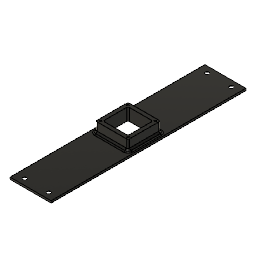
Foosball Table with Camera Stand (Autodesk Fusion 360 archive; units mm, degrees)
design "Camera Holder Middle"
Autodesk Fusion 360 part; units mm, degrees
note: some values were not read from the file. Chosen so that the rebuilt part matches the saved one: which bodies a step acts on; which face or edge a step refers to. Set by a fixed rule: which sketch regions a step uses.
(part 1 of 2)
sketch "Sketch1" plane through (0, 0, 0) normal (0, 0, 1) x (1, 0, 0)
  line L0 (-120.55, 25.4) -> (120.65, 25.4)
  line L1 (120.65, 25.4) -> (120.65, -25.4)
  line L2 (120.65, -25.4) -> (-120.55, -25.4)
  line L3 (-120.55, -25.4) -> (-120.55, 25.4)
  dimension "d3" = 241.2
  dimension "d4" = 50.8
  dimension "d5" = 25.4
  dimension "d6" = 120.65
  constraint horizontal L0
  constraint vertical L1
  constraint horizontal L2
  constraint vertical L3
  measures "d3" distance of L1 L3
  measures "d4" distance of L0 L2
  measures "d5" distance of origin L2
  measures "d6" distance of origin L1
extrude "Extrude1" add sketch "Sketch1" along normal blind 2.5
sketch "Sketch2" plane through (0, 0, 2.5) normal (0, 0, 1) x (-1, 0, 0)
  line L0 (120.55, 25.4) -> (-120.65, 25.4)
  line L1 (-120.65, 25.4) -> (-120.65, -25.4)
  line L2 (-120.65, -25.4) -> (120.55, -25.4)
  line L3 (120.55, -25.4) -> (120.55, 25.4)
  line L4 (13.4, -15.4) -> (-13.4, -15.4)
  line L5 (-15.4, -13.4) -> (-15.4, 13.4)
  line L6 (-13.4, 15.4) -> (13.4, 15.4)
  line L7 (15.4, 13.4) -> (15.4, -13.4)
  arc A0 (13.4, -15.4) -> (15.4, -13.4) centre (13.4, -13.4) ccw
  arc A1 (-15.4, -13.4) -> (-13.4, -15.4) centre (-13.4, -13.4) ccw
  arc A2 (-13.4, 15.4) -> (-15.4, 13.4) centre (-13.4, 13.4) ccw
  arc A3 (15.4, 13.4) -> (13.4, 15.4) centre (13.4, 13.4) ccw
  dimension "d7" = 30.8
  dimension "d8" = 30.8
  dimension "d9" = 15.4
  dimension "d10" = 15.4
  dimension "d11" = 2
  constraint horizontal L4
  constraint vertical L5
  constraint horizontal L6
  constraint vertical L7
  constraint tangent L4 A0
  constraint tangent L7 A0
  constraint tangent L4 A1
  constraint tangent L5 A1
  constraint equal A0 A1
  constraint tangent L5 A2
  constraint tangent L6 A2
  constraint equal A0 A2
  constraint tangent L6 A3
  constraint tangent L7 A3
  constraint equal A0 A3
  measures "d7" distance of L5 L7
  measures "d8" distance of L4 L6
  measures "d9" distance of origin L5
  measures "d10" distance of origin L4
  measures "d11" radius of A0
extrude "Extrude2" cut sketch "Sketch2" against normal blind 2.5 contours L4 L5 L6 L7 A0 A1 A2 A3
sketch "Sketch4" plane through (0, 0, 2.5) normal (0, 0, 1) x (-1, 0, 0)
  line L0 (15.4, 13.4) -> (15.4, -13.4)
  arc A0 (13.4, -15.4) -> (15.4, -13.4) centre (13.4, -13.4) ccw
  line L1 (13.4, -15.4) -> (-13.4, -15.4)
  arc A1 (-15.4, -13.4) -> (-13.4, -15.4) centre (-13.4, -13.4) ccw
  line L2 (-15.4, -13.4) -> (-15.4, 13.4)
  arc A2 (-13.4, 15.4) -> (-15.4, 13.4) centre (-13.4, 13.4) ccw
  line L3 (-13.4, 15.4) -> (13.4, 15.4)
  arc A3 (15.4, 13.4) -> (13.4, 15.4) centre (13.4, 13.4) ccw
  line L4 (120.55, 25.4) -> (-120.65, 25.4)
  line L5 (-120.65, 25.4) -> (-120.65, -25.4)
  line L6 (-120.65, -25.4) -> (120.55, -25.4)
  line L7 (120.55, -25.4) -> (120.55, 25.4)
  line L8 (18, -20) -> (-18, -20)
  line L9 (-20, -18) -> (-20, 18)
  line L10 (-18, 20) -> (18, 20)
  line L11 (20, 18) -> (20, -18)
  arc A4 (18, -20) -> (20, -18) centre (18, -18) ccw
  arc A5 (-20, -18) -> (-18, -20) centre (-18, -18) ccw
  arc A6 (-18, 20) -> (-20, 18) centre (-18, 18) ccw
  arc A7 (20, 18) -> (18, 20) centre (18, 18) ccw
  dimension "d18" = 40
  dimension "d19" = 40
  dimension "d20" = 20
  dimension "d21" = 20
  dimension "d22" = 2
  constraint horizontal L8
  constraint vertical L9
  constraint horizontal L10
  constraint vertical L11
  constraint tangent L8 A4
  constraint tangent L11 A4
  constraint tangent L8 A5
  constraint tangent L9 A5
  constraint equal A4 A5
  constraint tangent L9 A6
  constraint tangent L10 A6
  constraint equal A4 A6
  constraint tangent L10 A7
  constraint tangent L11 A7
  constraint equal A4 A7
  measures "d18" distance of L9 L11
  measures "d19" distance of L8 L10
  measures "d20" distance of origin L9
  measures "d21" distance of origin L8
  measures "d22" radius of A4
extrude "Extrude3" add sketch "Sketch4" along normal blind 2.5 contours L8 L9 L10 L11 A4 A5 A6 A7
sketch "Sketch6" plane through (0, 0, 5) normal (0, 0, 1) x (-1, 0, 0)
  arc A0 (13.4, -15.4) -> (15.4, -13.4) centre (13.4, -13.4) ccw
  line L0 (13.4, -15.4) -> (-13.4, -15.4)
  arc A1 (-15.4, -13.4) -> (-13.4, -15.4) centre (-13.4, -13.4) ccw
  line L1 (-15.4, -13.4) -> (-15.4, 13.4)
  arc A2 (-13.4, 15.4) -> (-15.4, 13.4) centre (-13.4, 13.4) ccw
  line L2 (-13.4, 15.4) -> (13.4, 15.4)
  arc A3 (15.4, 13.4) -> (13.4, 15.4) centre (13.4, 13.4) ccw
  line L3 (15.4, 13.4) -> (15.4, -13.4)
  arc A4 (18, -20) -> (20, -18) centre (18, -18) ccw
  line L4 (20, -18) -> (20, 18)
  arc A5 (20, 18) -> (18, 20) centre (18, 18) ccw
  line L5 (18, 20) -> (-18, 20)
  arc A6 (-18, 20) -> (-20, 18) centre (-18, 18) ccw
  line L6 (-20, 18) -> (-20, -18)
  arc A7 (-20, -18) -> (-18, -20) centre (-18, -18) ccw
  line L7 (-18, -20) -> (18, -20)
  point P0 (17, -17)
  point P1 (-17, -17)
  point P2 (-17, 17)
  point P3 (17, 17)
  dimension "d29" = 34
  dimension "d30" = 34
  dimension "d31" = 17
  dimension "d32" = 17
  constraint horizontal P0 P1
  constraint vertical P1 P2
  constraint horizontal P2 P3
  constraint vertical P0 P3
  measures "d29" horizontal distance of P0 P1
  measures "d30" vertical distance of P1 P2
  measures "d31" horizontal distance of origin P1
  measures "d32" vertical distance of origin P1
hole "Hole1" at (-17, 17, 5) at (17, 17, 5) at (17, -17, 5) at (-17, -17, 5) direction (0, 0, -1) diameter 2.54 depth 5 tip angle 118
chamfer "Chamfer1" distance 2.5 distance2 2.5 8 edges at (0, -20, 2.5) (-19.4142, -19.4142, 2.5) (-20, 0, 2.5) (-19.4142, 19.4142, 2.5) (0, 20, 2.5) (19.4142, 19.4142, 2.5) (20, 0, 2.5) (19.4142, -19.4142, 2.5) measured on face at (87.1, -6, 2.5) measured on face at (87.1, -6, 2.5) measured on face at (87.1, -6, 2.5) measured on face at (87.1, -6, 2.5) measured on face at (87.1, -6, 2.5) measured on face at (87.1, -6, 2.5) measured on face at (87.1, -6, 2.5) measured on face at (87.1, -6, 2.5)
fillet "Fillet1" radius 2.5 8 edges at (22.5, 0, 2.5) (21.182, 21.182, 2.5) (0, 22.5, 2.5) (-21.182, 21.182, 2.5) (-22.5, 0, 2.5) (-21.182, -21.182, 2.5) (0, -22.5, 2.5) (21.182, -21.182, 2.5)
sketch "Sketch7" plane through (0, 0, 0) normal (0, 0, -1) x (1, 0, 0)
  circle A0 centre (17, 17) radius 1.27
  circle A1 centre (-17, -17) radius 1.27
  circle A2 centre (17, -17) radius 1.27
  circle A3 centre (-17, 17) radius 1.27
  line L0 (-15.4, -13.4) -> (-15.4, 13.4)
  arc A4 (-13.4, 15.4) -> (-15.4, 13.4) centre (-13.4, 13.4) ccw
  line L1 (-13.4, 15.4) -> (13.4, 15.4)
  arc A5 (15.4, 13.4) -> (13.4, 15.4) centre (13.4, 13.4) ccw
  line L2 (15.4, 13.4) -> (15.4, -13.4)
  arc A6 (13.4, -15.4) -> (15.4, -13.4) centre (13.4, -13.4) ccw
  line L3 (13.4, -15.4) -> (-13.4, -15.4)
  arc A7 (-15.4, -13.4) -> (-13.4, -15.4) centre (-13.4, -13.4) ccw
  line L4 (120.65, 25.4) -> (-120.55, 25.4)
  line L5 (-120.55, 25.4) -> (-120.55, -25.4)
  line L6 (-120.55, -25.4) -> (120.65, -25.4)
  line L7 (120.65, -25.4) -> (120.65, 25.4)
  point P0 (-112.9, 15)
  point P1 (-112.9, -15)
  point P2 (113, 15)
  point P3 (113, -15)
  dimension "d40" = 30
  dimension "d41" = 7.65
  dimension "d42" = 7.65
  dimension "d48" = 10.4
  constraint horizontal P0 P2
  constraint vertical P2 P3
  constraint horizontal P1 P3
  constraint vertical P0 P1
  measures "d40" distance of P0 P1
  measures "d41" distance of L5 P0
  measures "d42" distance of L7 P2
  measures "d48" distance of L4 P0
hole "Hole2" at (-112.9, -15, 0) at (-112.9, 15, 0) at (113, -15, 0) at (113, 15, 0) direction (0, 0, 1) diameter 4.5 depth 5 tip angle 180 countersink diameter 9.4 countersink angle 90
extrude "Extrude5" add 1 faces at (-17.0425, 4.4667, 5) along direction (0, 0, 1) blind 10
equation "d3 = 9.5 in - 0.1 mm"
equation "d6 = ( 9.5 / 2 ) * 1 in"
equation "d41 = ( ( 15.4 / 2 ) * 1 mm ) - 0.05 * 1 mm"
equation "d42 = ( ( 15.4 / 2 ) * 1 mm ) - 0.05 * 1 mm"
equation "d48 = ( 2 in - 30 mm ) / 2"

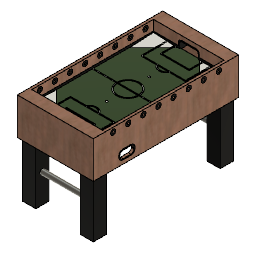
design "Foosball Table"
Autodesk Fusion 360 part; units mm, degrees
sketch "Sketch1" plane through (0, 0, 0) normal (0, 0, 1) x (1, 0, 0)
  line L0 (-365, 698.5) -> (365, 698.5)
  line L1 (365, 698.5) -> (365, -698.5)
  line L2 (365, -698.5) -> (-365, -698.5)
  line L3 (-365, -698.5) -> (-365, 698.5)
  dimension "d1" = 1397
  dimension "d2" = 730
  dimension "d3" = 365
  dimension "d4" = 698.5
  constraint horizontal L0
  constraint vertical L1
  constraint horizontal L2
  constraint vertical L3
  measures "d1" distance of L0 L2
  measures "d2" distance of L1 L3
  measures "d3" distance of origin L3
  measures "d4" distance of origin L0
extrude "Extrude1" add sketch "Sketch1" along normal blind 355.6 makes body 1
sketch "Sketch2" plane through (0, 0, 355.6) normal (0, 0, 1) x (-1, 0, 0)
  line L0 (365, 698.5) -> (-365, 698.5)
  line L1 (-365, 698.5) -> (-365, -698.5)
  line L2 (-365, -698.5) -> (365, -698.5)
  line L3 (365, -698.5) -> (365, 698.5)
  line L4 (339.6, 584.2) -> (-339.6, 584.2)
  line L5 (-339.6, 584.2) -> (-339.6, -584.2)
  line L6 (-339.6, -584.2) -> (339.6, -584.2)
  line L7 (339.6, -584.2) -> (339.6, 584.2)
  dimension "d7" = 25.4
  dimension "d8" = 25.4
  dimension "d9" = 114.3
  dimension "d10" = 114.3
  constraint horizontal L4
  constraint vertical L5
  constraint horizontal L6
  constraint vertical L7
  measures "d7" distance of L3 L7
  measures "d8" distance of L1 L5
  measures "d9" distance of L0 L4
  measures "d10" distance of L2 L6
extrude "Extrude2" cut sketch "Sketch2" along normal blind 0 and the other way blind 118 contours L4 L5 L6 L7 bodies 1
sketch "Sketch3" plane through (0, 0, 0) normal (0, 0, -1) x (1, 0, 0)
  line L0 (365, 698.5) -> (-365, 698.5)
  line L1 (-365, 698.5) -> (-365, -698.5)
  line L2 (-365, -698.5) -> (365, -698.5)
  line L3 (365, -698.5) -> (365, 698.5)
  line L4 (339.6, 673.1) -> (212.6, 673.1)
  line L5 (212.6, 673.1) -> (212.6, 546.1)
  line L6 (212.6, 546.1) -> (339.6, 546.1)
  line L7 (339.6, 546.1) -> (339.6, 673.1)
  line L8 (-212.6, 673.1) -> (-339.6, 673.1)
  line L9 (-339.6, 673.1) -> (-339.6, 546.1)
  line L10 (-339.6, 546.1) -> (-212.6, 546.1)
  line L11 (-212.6, 546.1) -> (-212.6, 673.1)
  line L12 (339.6, -546.1) -> (212.6, -546.1)
  line L13 (212.6, -546.1) -> (212.6, -673.1)
  line L14 (212.6, -673.1) -> (339.6, -673.1)
  line L15 (339.6, -673.1) -> (339.6, -546.1)
  line L16 (-212.6, -546.1) -> (-339.6, -546.1)
  line L17 (-339.6, -546.1) -> (-339.6, -673.1)
  line L18 (-339.6, -673.1) -> (-212.6, -673.1)
  line L19 (-212.6, -673.1) -> (-212.6, -546.1)
  dimension "d15" = 127
  dimension "d16" = 127
  dimension "d17" = 25.4
  dimension "d18" = 25.4
  dimension "d19" = 127
  dimension "d20" = 127
  dimension "d21" = 25.4
  dimension "d22" = 25.4
  dimension "d23" = 127
  dimension "d24" = 127
  dimension "d25" = 25.4
  dimension "d26" = 25.4
  dimension "d27" = 127
  dimension "d28" = 127
  dimension "d29" = 25.4
  dimension "d30" = 25.4
  constraint horizontal L4
  constraint vertical L5
  constraint horizontal L6
  constraint vertical L7
  constraint horizontal L8
  constraint vertical L9
  constraint horizontal L10
  constraint vertical L11
  constraint horizontal L12
  constraint vertical L13
  constraint horizontal L14
  constraint vertical L15
  constraint horizontal L16
  constraint vertical L17
  constraint horizontal L18
  constraint vertical L19
  measures "d15" distance of L4 L6
  measures "d16" distance of L5 L7
  measures "d17" distance of L3 L7
  measures "d18" distance of L0 L4
  measures "d19" distance of L8 L10
  measures "d20" distance of L9 L11
  measures "d21" distance of L1 L9
  measures "d22" distance of L0 L8
  measures "d23" distance of L13 L15
  measures "d24" distance of L12 L14
  measures "d25" distance of L3 L15
  measures "d26" distance of L2 L14
  measures "d27" distance of L17 L19
  measures "d28" distance of L16 L18
  measures "d29" distance of L2 L18
  measures "d30" distance of L1 L17
extrude "Extrude3" add sketch "Sketch3" along normal blind 529.4 contours L4 L5 L6 L7 | L8 L9 L10 L11 | L12 L13 L14 L15 | L16 L17 L18 L19 bodies 1
sketch "Sketch4" plane through (-212.6, 0, 0) normal (1, 0, 0) x (0, 1, 0)
  line L0 (-546.1, 0) -> (-673.1, 0)
  line L1 (-673.1, 0) -> (-673.1, -529.4)
  line L2 (-673.1, -529.4) -> (-546.1, -529.4)
  line L3 (-546.1, -529.4) -> (-546.1, 0)
  circle A0 centre (-609.6, -249.6) radius 25
  circle A1 centre (609.6, -249.6) radius 25
  line L4 (673.1, 0) -> (673.1, -529.4)
  line L5 (673.1, -529.4) -> (546.1, -529.4)
  dimension "d33" = 50
  dimension "d34" = 63.5
  dimension "d35" = 279.8
  dimension "d36" = 50
  dimension "d37" = 63.5
  dimension "d38" = 279.8
  measures "d33" diameter of A0
  measures "d34" distance of L1 A0.centre
  measures "d35" distance of L2 A0.centre
  measures "d36" diameter of A1
  measures "d37" distance of A1.centre L4
  measures "d38" distance of A1.centre L5
extrude "Extrude4" add sketch "Sketch4" along normal blind 425.2 contours A0 | A1 bodies 1
sketch "Sketch5" plane through (365, 0, 0) normal (1, 0, 0) x (0, 1, 0)
  line L0 (-698.5, 0) -> (698.5, 0)
  line L1 (698.5, 0) -> (698.5, 355.6)
  line L2 (698.5, 355.6) -> (-698.5, 355.6)
  line L3 (-698.5, 355.6) -> (-698.5, 0)
  circle A0 centre (507.5, 315.6) radius 8.75
  circle A1 centre (362.5, 315.6) radius 8.75
  circle A2 centre (217.5, 315.6) radius 8.75
  circle A3 centre (72.5, 315.6) radius 8.75
  circle A4 centre (-72.5, 315.6) radius 8.75
  circle A5 centre (-217.5, 315.6) radius 8.75
  circle A6 centre (-362.5, 315.6) radius 8.75
  circle A7 centre (-507.5, 315.6) radius 8.75
  dimension "d41" = 17.5
  dimension "d42" = 17.5
  dimension "d43" = 17.5
  dimension "d44" = 17.5
  dimension "d45" = 17.5
  dimension "d46" = 17.5
  dimension "d47" = 17.5
  dimension "d48" = 17.5
  dimension "d49" = 145
  dimension "d50" = 145
  dimension "d51" = 145
  dimension "d52" = 145
  dimension "d53" = 145
  dimension "d54" = 145
  dimension "d55" = 145
  dimension "d56" = 191
  dimension "d57" = 40
  constraint horizontal A0.centre A1.centre
  constraint horizontal A1.centre A2.centre
  constraint horizontal A3.centre A2.centre
  constraint horizontal A3.centre A4.centre
  constraint horizontal A5.centre A4.centre
  constraint horizontal A6.centre A5.centre
  constraint horizontal A7.centre A6.centre
  measures "d41" diameter of A0
  measures "d42" diameter of A1
  measures "d43" diameter of A2
  measures "d44" diameter of A3
  measures "d45" diameter of A4
  measures "d46" diameter of A5
  measures "d47" diameter of A6
  measures "d48" diameter of A7
  measures "d49" distance of A0.centre A1.centre
  measures "d50" distance of A1.centre A2.centre
  measures "d51" distance of A3.centre A2.centre
  measures "d52" distance of A3.centre A4.centre
  measures "d53" distance of A5.centre A4.centre
  measures "d54" distance of A6.centre A5.centre
  measures "d55" distance of A7.centre A6.centre
  measures "d56" distance of L1 A0.centre
  measures "d57" distance of L2 A7.centre
extrude "Extrude5" cut sketch "Sketch5" against normal blind 730 contours A0 | A1 | A2 | A3 | A4 | A5 | A6 | A7 bodies 1
sketch "Sketch6" plane through (365, 0, 0) normal (1, 0, 0) x (0, 1, 0)
  circle A0 centre (217.5, 315.6) radius 8.75
  circle A1 centre (-362.5, 315.6) radius 8.75
  circle A2 centre (-217.5, 315.6) radius 8.75
  circle A3 centre (362.5, 315.6) radius 8.75
  circle A4 centre (72.5, 315.6) radius 8.75
  circle A5 centre (-507.5, 315.6) radius 8.75
  circle A6 centre (-72.5, 315.6) radius 8.75
  circle A7 centre (507.5, 315.6) radius 8.75
  line L0 (-698.5, 0) -> (698.5, 0)
  line L1 (698.5, 0) -> (698.5, 355.6)
  line L2 (698.5, 355.6) -> (-698.5, 355.6)
  line L3 (-698.5, 355.6) -> (-698.5, 0)
  circle A8 centre (-507.5, 315.6) radius 25
  circle A9 centre (-362.5, 315.6) radius 25
  circle A10 centre (-217.5, 315.6) radius 25
  circle A11 centre (-72.5, 315.6) radius 25
  circle A12 centre (72.5, 315.6) radius 25
  circle A13 centre (217.5, 315.6) radius 25
  circle A14 centre (362.5, 315.6) radius 25
  circle A15 centre (507.5, 315.6) radius 25
  dimension "d60" = 50
  dimension "d61" = 50
  dimension "d62" = 50
  dimension "d63" = 50
  dimension "d64" = 50
  dimension "d65" = 50
  dimension "d66" = 50
  dimension "d67" = 50
  constraint concentric A5 A8
  constraint concentric A1 A9
  constraint concentric A2 A10
  constraint concentric A6 A11
  constraint concentric A4 A12
  constraint concentric A0 A13
  constraint concentric A3 A14
  constraint concentric A7 A15
  measures "d60" diameter of A8
  measures "d61" diameter of A9
  measures "d62" diameter of A10
  measures "d63" diameter of A11
  measures "d64" diameter of A12
  measures "d65" diameter of A13
  measures "d66" diameter of A14
  measures "d67" diameter of A15
extrude "Extrude6" add sketch "Sketch6" along normal blind 1 contours A8 | A9 | A10 | A11 | A12 | A13 | A14 | A15 bodies 1
sketch "Sketch7" plane through (-365, 0, 0) normal (-1, 0, 0) x (0, -1, 0)
  circle A0 centre (-217.5, 315.6) radius 8.75
  circle A1 centre (362.5, 315.6) radius 8.75
  circle A2 centre (217.5, 315.6) radius 8.75
  circle A3 centre (-362.5, 315.6) radius 8.75
  circle A4 centre (-72.5, 315.6) radius 8.75
  circle A5 centre (507.5, 315.6) radius 8.75
  circle A6 centre (72.5, 315.6) radius 8.75
  circle A7 centre (-507.5, 315.6) radius 8.75
  line L0 (-698.5, 0) -> (698.5, 0)
  line L1 (698.5, 0) -> (698.5, 355.6)
  line L2 (698.5, 355.6) -> (-698.5, 355.6)
  line L3 (-698.5, 355.6) -> (-698.5, 0)
  circle A8 centre (-507.5, 315.6) radius 25
  circle A9 centre (-362.5, 315.6) radius 25
  circle A10 centre (-217.5, 315.6) radius 25
  circle A11 centre (-72.5, 315.6) radius 25
  circle A12 centre (72.5, 315.6) radius 25
  circle A13 centre (217.5, 315.6) radius 25
  circle A14 centre (362.5, 315.6) radius 25
  circle A15 centre (507.5, 315.6) radius 25
  dimension "d70" = 50
  dimension "d71" = 50
  dimension "d72" = 50
  dimension "d73" = 50
  dimension "d74" = 50
  dimension "d75" = 50
  dimension "d76" = 50
  dimension "d77" = 50
  constraint concentric A7 A8
  constraint concentric A3 A9
  constraint concentric A0 A10
  constraint concentric A4 A11
  constraint concentric A6 A12
  constraint concentric A2 A13
  constraint concentric A1 A14
  constraint concentric A5 A15
  measures "d70" diameter of A8
  measures "d71" diameter of A9
  measures "d72" diameter of A10
  measures "d73" diameter of A11
  measures "d74" diameter of A12
  measures "d75" diameter of A13
  measures "d76" diameter of A14
  measures "d77" diameter of A15
extrude "Extrude7" add sketch "Sketch7" along normal blind 1 contours A8 | A9 | A10 | A11 | A12 | A13 | A14 | A15 bodies 1
sketch "Sketch10" plane through (0, 0, 0) normal (0, 0, -1) x (1, 0, 0)
  line L0 (-212.6, 546.1) -> (-339.6, 546.1)
  line L1 (-339.6, 546.1) -> (-339.6, 673.1)
  line L2 (-339.6, 673.1) -> (-212.6, 673.1)
  line L3 (-212.6, 673.1) -> (-212.6, 546.1)
  line L4 (339.6, 546.1) -> (212.6, 546.1)
  line L5 (212.6, 546.1) -> (212.6, 673.1)
  line L6 (212.6, 673.1) -> (339.6, 673.1)
  line L7 (339.6, 673.1) -> (339.6, 546.1)
  line L8 (-212.6, -673.1) -> (-339.6, -673.1)
  line L9 (-339.6, -673.1) -> (-339.6, -546.1)
  line L10 (-339.6, -546.1) -> (-212.6, -546.1)
  line L11 (-212.6, -546.1) -> (-212.6, -673.1)
  line L12 (339.6, -673.1) -> (212.6, -673.1)
  line L13 (212.6, -673.1) -> (212.6, -546.1)
  line L14 (212.6, -546.1) -> (339.6, -546.1)
  line L15 (339.6, -546.1) -> (339.6, -673.1)
  line L16 (365, 698.5) -> (-365, 698.5)
  line L17 (-365, 698.5) -> (-365, -698.5)
  line L18 (-365, -698.5) -> (365, -698.5)
  line L19 (365, -698.5) -> (365, 698.5)
  line L20 (339.6, -673.1) -> (-339.6, -673.1)
  line L21 (-339.6, -673.1) -> (-339.6, 673.1)
  line L22 (-339.6, 673.1) -> (339.6, 673.1)
  line L23 (339.6, 673.1) -> (339.6, -673.1)
  constraint horizontal L20
  constraint vertical L21
  constraint horizontal L22
  constraint vertical L23
  constraint coincident L1 L2.start
  constraint coincident L12.start L15.end
  constraint horizontal L6.end L1.end
extrude "Extrude8" cut sketch "Sketch10" against normal blind 227.6 contours L0 L3 L4 L5 L10 L11 L13 L14 L20 L21 L22 L23 bodies 1
sketch "Sketch8" plane through (365, 0, 0) normal (1, 0, 0) x (0, 1, 0)
  circle A0 centre (507.5, 315.6) radius 25
  circle A1 centre (-72.5, 315.6) radius 25
  circle A2 centre (-507.5, 315.6) radius 25
  circle A3 centre (72.5, 315.6) radius 25
  circle A4 centre (362.5, 315.6) radius 25
  circle A5 centre (-217.5, 315.6) radius 25
  circle A6 centre (-362.5, 315.6) radius 25
  circle A7 centre (217.5, 315.6) radius 25
  line L0 (-698.5, 0) -> (698.5, 0)
  line L1 (698.5, 0) -> (698.5, 355.6)
  line L2 (698.5, 355.6) -> (-698.5, 355.6)
  line L3 (-698.5, 355.6) -> (-698.5, 0)
  line L4 (-413.5, 117.5) -> (-338.5, 117.5)
  line L5 (-308.5, 87.5) -> (-308.5, 77.5)
  line L6 (-338.5, 47.5) -> (-413.5, 47.5)
  line L7 (-443.5, 77.5) -> (-443.5, 87.5)
  arc A8 (-413.5, 117.5) -> (-443.5, 87.5) centre (-413.5, 87.5) ccw
  arc A9 (-443.5, 77.5) -> (-413.5, 47.5) centre (-413.5, 77.5) ccw
  arc A10 (-338.5, 47.5) -> (-308.5, 77.5) centre (-338.5, 77.5) ccw
  arc A11 (-308.5, 87.5) -> (-338.5, 117.5) centre (-338.5, 87.5) ccw
  line L8 (-413.5, 127.5) -> (-338.5, 127.5)
  line L9 (-298.5, 87.5) -> (-298.5, 77.5)
  line L10 (-338.5, 37.5) -> (-413.5, 37.5)
  line L11 (-453.5, 77.5) -> (-453.5, 87.5)
  arc A12 (-413.5, 127.5) -> (-453.5, 87.5) centre (-413.5, 87.5) ccw
  arc A13 (-453.5, 77.5) -> (-413.5, 37.5) centre (-413.5, 77.5) ccw
  arc A14 (-338.5, 37.5) -> (-298.5, 77.5) centre (-338.5, 77.5) ccw
  arc A15 (-298.5, 87.5) -> (-338.5, 127.5) centre (-338.5, 87.5) ccw
  dimension "d80" = 47.5
  dimension "d81" = 70
  dimension "d82" = 255
  dimension "d83" = 135
  dimension "d84" = 30
  dimension "d92" = 10
  dimension "d93" = 10
  dimension "d94" = 10
  dimension "d95" = 10
  dimension "d96" = 40
  constraint horizontal L4
  constraint vertical L5
  constraint horizontal L6
  constraint vertical L7
  constraint tangent L4 A8
  constraint tangent L7 A8
  constraint tangent L7 A9
  constraint tangent L6 A9
  constraint equal A8 A9
  constraint tangent L6 A10
  constraint tangent L5 A10
  constraint equal A8 A10
  constraint tangent L5 A11
  constraint tangent L4 A11
  constraint equal A8 A11
  constraint horizontal L8
  constraint vertical L9
  constraint horizontal L10
  constraint vertical L11
  constraint tangent L8 A12
  constraint tangent L11 A12
  constraint tangent L11 A13
  constraint tangent L10 A13
  constraint equal A12 A13
  constraint tangent L9 A14
  constraint tangent L10 A14
  constraint equal A12 A14
  constraint tangent L9 A15
  constraint tangent L8 A15
  constraint equal A12 A15
  measures "d45" diameter of L0.end
  measures "d63" diameter of L0.end
  measures "d74" diameter of L0.end
  measures "d80" distance of L0 L6
  measures "d81" distance of L4 L6
  measures "d82" distance of L3 L7
  measures "d83" distance of L5 L7
  measures "d84" radius of A8
  measures "d92" distance of L4 L8
  measures "d93" distance of L6 L10
  measures "d94" distance of L5 L9
  measures "d95" distance of L7 L11
  measures "d96" radius of A12
  measures "d237" diameter of L0.end
  measures "d248" diameter of L0.end
extrude "Extrude9" cut sketch "Sketch8" against normal blind 25.4 contours L4 L5 L6 L7 A8 A9 A10 A11 bodies 1
extrude "Extrude10" add sketch "Sketch8" along normal blind 1 contours L8 L9 L10 L11 A12 A13 A14 A15 bodies 1
sketch "Sketch11" plane through (-365, 0, 0) normal (-1, 0, 0) x (0, -1, 0)
  circle A0 centre (507.5, 315.6) radius 25
  circle A1 centre (-72.5, 315.6) radius 25
  circle A2 centre (-507.5, 315.6) radius 25
  circle A3 centre (72.5, 315.6) radius 25
  circle A4 centre (362.5, 315.6) radius 25
  circle A5 centre (-217.5, 315.6) radius 25
  circle A6 centre (-362.5, 315.6) radius 25
  circle A7 centre (217.5, 315.6) radius 25
  line L0 (-698.5, 0) -> (698.5, 0)
  line L1 (698.5, 0) -> (698.5, 355.6)
  line L2 (698.5, 355.6) -> (-698.5, 355.6)
  line L3 (-698.5, 355.6) -> (-698.5, 0)
  line L4 (-413.5, 127.5) -> (-338.5, 127.5)
  line L5 (-298.5, 87.5) -> (-298.5, 77.5)
  line L6 (-338.5, 37.5) -> (-413.5, 37.5)
  line L7 (-453.5, 77.5) -> (-453.5, 87.5)
  line L8 (-413.5, 117.5) -> (-338.5, 117.5)
  line L9 (-308.5, 87.5) -> (-308.5, 77.5)
  line L10 (-338.5, 47.5) -> (-413.5, 47.5)
  line L11 (-443.5, 77.5) -> (-443.5, 87.5)
  arc A8 (-413.5, 117.5) -> (-443.5, 87.5) centre (-413.5, 87.5) ccw
  arc A9 (-443.5, 77.5) -> (-413.5, 47.5) centre (-413.5, 77.5) ccw
  arc A10 (-338.5, 47.5) -> (-308.5, 77.5) centre (-338.5, 77.5) ccw
  arc A11 (-308.5, 87.5) -> (-338.5, 117.5) centre (-338.5, 87.5) ccw
  arc A12 (-413.5, 127.5) -> (-453.5, 87.5) centre (-413.5, 87.5) ccw
  arc A13 (-453.5, 77.5) -> (-413.5, 37.5) centre (-413.5, 77.5) ccw
  arc A14 (-338.5, 37.5) -> (-298.5, 77.5) centre (-338.5, 77.5) ccw
  arc A15 (-298.5, 87.5) -> (-338.5, 127.5) centre (-338.5, 87.5) ccw
  dimension "d101" = 10
  dimension "d102" = 10
  dimension "d103" = 10
  dimension "d104" = 10
  dimension "d106" = 70
  dimension "d107" = 245
  dimension "d108" = 37.5
  dimension "d109" = 135
  dimension "d110" = 30
  dimension "d111" = 40
  constraint horizontal L4
  constraint vertical L5
  constraint horizontal L6
  constraint vertical L7
  constraint horizontal L8
  constraint vertical L9
  constraint horizontal L10
  constraint vertical L11
  constraint tangent L8 A8
  constraint tangent L11 A8
  constraint tangent L11 A9
  constraint tangent L10 A9
  constraint equal A8 A9
  constraint tangent L10 A10
  constraint tangent L9 A10
  constraint equal A8 A10
  constraint tangent L9 A11
  constraint tangent L8 A11
  constraint equal A8 A11
  constraint tangent L4 A12
  constraint tangent L7 A12
  constraint tangent L7 A13
  constraint tangent L6 A13
  constraint equal A12 A13
  constraint tangent L6 A14
  constraint tangent L5 A14
  constraint equal A12 A14
  constraint tangent L5 A15
  constraint tangent L4 A15
  constraint equal A12 A15
  measures "d101" distance of L6 L10
  measures "d102" distance of L7 L11
  measures "d103" distance of L4 L8
  measures "d104" distance of L5 L9
  measures "d106" distance of L8 L10
  measures "d107" distance of L3 L7
  measures "d108" distance of L0 L6
  measures "d109" distance of L9 L11
  measures "d110" radius of A8
  measures "d111" radius of A12
extrude "Extrude11" cut sketch "Sketch11" against normal blind 25.4 contours L8 L9 L10 L11 A8 A9 A10 A11 bodies 1
extrude "Extrude12" add sketch "Sketch11" along normal blind 1 contours L4 L5 L6 L7 A12 A13 A14 A15 bodies 1
sketch "Sketch12" plane through (0, 0, 237.6) normal (0, 0, 1) x (-1, 0, 0)
  line L0 (339.6, -584.2) -> (339.6, 584.2)
  line L1 (339.6, 584.2) -> (-339.6, 584.2)
  line L2 (-339.6, 584.2) -> (-339.6, -584.2)
  line L3 (-339.6, -584.2) -> (339.6, -584.2)
  line L4 (339.6, 5) -> (-339.6, 5)
  line L5 (-339.6, 5) -> (-339.6, -5)
  line L6 (-339.6, -5) -> (339.6, -5)
  line L7 (339.6, -5) -> (339.6, 5)
  dimension "d116" = 10
  dimension "d117" = 5
  constraint horizontal L4
  constraint vertical L5
  constraint horizontal L6
  constraint vertical L7
  constraint coincident L2 L5.end
  constraint coincident L0 L4.start
  measures "d116" distance of L4 L6
  measures "d117" distance of origin L6
split_face "SplitFace1" 1 faces at (-113.2, 194.7333, 237.6) by curves path "Sketch12" along L6 L7 L4 L5 on bodies 1
sketch "Sketch13" plane through (0, 584.2, 0) normal (0, -1, 0) x (1, 0, 0)
  line L0 (339.6, 355.6) -> (-339.6, 355.6)
  line L1 (-339.6, 355.6) -> (-339.6, 237.6)
  line L2 (-339.6, 237.6) -> (339.6, 237.6)
  line L3 (339.6, 237.6) -> (339.6, 355.6)
  line L4 (-70, 305.1) -> (70, 305.1)
  line L5 (90, 285.1) -> (90, 237.6)
  line L6 (90, 237.6) -> (-90, 237.6)
  line L7 (-90, 237.6) -> (-90, 285.1)
  arc A0 (-70, 305.1) -> (-90, 285.1) centre (-70, 285.1) ccw
  arc A1 (90, 285.1) -> (70, 305.1) centre (70, 285.1) ccw
  line L8 (-70, 315.1) -> (70, 315.1)
  line L9 (100, 285.1) -> (100, 237.6)
  line L10 (100, 237.6) -> (-100, 237.6)
  line L11 (-100, 237.6) -> (-100, 285.1)
  arc A2 (-70, 315.1) -> (-100, 285.1) centre (-70, 285.1) ccw
  arc A3 (100, 285.1) -> (70, 315.1) centre (70, 285.1) ccw
  dimension "d118" = 180
  dimension "d119" = 67.5
  dimension "d120" = 90
  dimension "d121" = 20
  dimension "d122" = 200
  dimension "d123" = 100
  dimension "d124" = 10
  dimension "d125" = 30
  constraint horizontal L4
  constraint vertical L5
  constraint horizontal L6
  constraint vertical L7
  constraint horizontal L1.end L6.end
  constraint tangent L4 A0
  constraint tangent L7 A0
  constraint tangent L4 A1
  constraint tangent L5 A1
  constraint equal A0 A1
  constraint horizontal L8
  constraint vertical L9
  constraint horizontal L10
  constraint vertical L11
  constraint coincident L2 L9.end
  constraint tangent L8 A2
  constraint tangent L11 A2
  constraint tangent L8 A3
  constraint tangent L9 A3
  constraint equal A2 A3
  measures "d118" distance of L5 L7
  measures "d119" distance of L4 L6
  measures "d120" distance of origin L7
  measures "d121" radius of A0
  measures "d122" distance of L9 L11
  measures "d123" distance of origin L11
  measures "d124" distance of L4 L8
  measures "d125" radius of A2
extrude "Extrude13" cut sketch "Sketch13" against normal blind 88.9 contours L2 L4 L5 L6 L7 A0 A1 L10 bodies 1
extrude "Extrude14" add sketch "Sketch13" along normal blind 1 contours L2 L4 L5 L7 A0 A1 L8 L9 L10 L11 A2 A3 bodies 1
sketch "Sketch14" plane through (0, -584.2, 0) normal (0, 1, 0) x (-1, 0, 0)
  line L0 (339.6, 355.6) -> (-339.6, 355.6)
  line L1 (-339.6, 355.6) -> (-339.6, 237.6)
  line L2 (-339.6, 237.6) -> (339.6, 237.6)
  line L3 (339.6, 237.6) -> (339.6, 355.6)
  line L4 (-70, 305.1) -> (70, 305.1)
  line L5 (90, 285.1) -> (90, 237.6)
  line L6 (90, 237.6) -> (-90, 237.6)
  line L7 (-90, 237.6) -> (-90, 285.1)
  line L8 (-70, 315.1) -> (70, 315.1)
  line L9 (100, 285.1) -> (100, 237.6)
  line L10 (100, 237.6) -> (-100, 237.6)
  line L11 (-100, 237.6) -> (-100, 285.1)
  arc A0 (-70, 305.1) -> (-90, 285.1) centre (-70, 285.1) ccw
  arc A1 (90, 285.1) -> (70, 305.1) centre (70, 285.1) ccw
  arc A2 (-70, 315.1) -> (-100, 285.1) centre (-70, 285.1) ccw
  arc A3 (100, 285.1) -> (70, 315.1) centre (70, 285.1) ccw
  dimension "d130" = 180
  dimension "d131" = 90
  dimension "d132" = 67.5
  dimension "d133" = 200
  dimension "d134" = 100
  dimension "d135" = 10
  dimension "d136" = 20
  dimension "d137" = 30
  constraint horizontal L4
  constraint vertical L5
  constraint horizontal L6
  constraint vertical L7
  constraint coincident L2 L5.end
  constraint horizontal L8
  constraint vertical L9
  constraint horizontal L10
  constraint vertical L11
  constraint coincident L2 L9.end
  constraint tangent L4 A0
  constraint tangent L7 A0
  constraint tangent L4 A1
  constraint tangent L5 A1
  constraint equal A0 A1
  constraint tangent L8 A2
  constraint tangent L11 A2
  constraint tangent L8 A3
  constraint tangent L9 A3
  constraint equal A2 A3
  measures "d130" distance of L5 L7
  measures "d131" distance of origin L7
  measures "d132" distance of L4 L6
  measures "d133" distance of L9 L11
  measures "d134" distance of origin L11
  measures "d135" distance of L4 L8
  measures "d136" radius of A0
  measures "d137" radius of A2
extrude "Extrude15" cut sketch "Sketch14" against normal blind 88.9 contours L2 L4 L5 L6 L7 L10 A0 A1 bodies 1
extrude "Extrude16" add sketch "Sketch14" along normal blind 1 contours L2 L4 L5 L7 L8 L9 L10 L11 A0 A1 A2 A3 bodies 1
sketch "Sketch15" plane through (0, -584.2, 0) normal (0, 1, 0) x (-1, 0, 0)
  line L0 (-100, 237.6) -> (-100, 285.1)
  arc A0 (-70, 315.1) -> (-100, 285.1) centre (-70, 285.1) ccw
  line L1 (-70, 315.1) -> (70, 315.1)
  arc A1 (100, 285.1) -> (70, 315.1) centre (70, 285.1) ccw
  line L2 (100, 285.1) -> (100, 237.6)
  line L3 (100, 237.6) -> (339.6, 237.6)
  line L4 (339.6, 237.6) -> (339.6, 355.6)
  line L5 (339.6, 355.6) -> (-339.6, 355.6)
  line L6 (-339.6, 355.6) -> (-339.6, 237.6)
  line L7 (-339.6, 237.6) -> (-100, 237.6)
  line L8 (-100, 237.6) -> (-339.6, 237.6)
  line L9 (-339.6, 237.6) -> (-339.6, 257.6)
  line L10 (-339.6, 257.6) -> (-100, 257.6)
  line L11 (-100, 257.6) -> (-100, 237.6)
  line L12 (100, 237.6) -> (339.6, 237.6)
  line L13 (339.6, 237.6) -> (339.6, 257.6)
  line L14 (339.6, 257.6) -> (100, 257.6)
  line L15 (100, 257.6) -> (100, 237.6)
  dimension "d142" = 20
  dimension "d143" = 20
  constraint horizontal L8
  constraint vertical L9
  constraint horizontal L10
  constraint vertical L11
  constraint coincident L6 L9.end
  constraint coincident L0.start L7.end
  constraint horizontal L12
  constraint vertical L13
  constraint horizontal L14
  constraint vertical L15
  constraint coincident L4 L13.end
  constraint coincident L2.end L3.start
  measures "d142" distance of L12 L14
  measures "d143" distance of L8 L10
extrude "Extrude17" add sketch "Sketch15" along normal blind 1 contours L0 L6 L7 L8 L9 L10 L11 | L2 L3 L4 L12 L13 L14 L15 bodies 1
sketch "Sketch16" plane through (0, 584.2, 0) normal (0, -1, 0) x (1, 0, 0)
  line L0 (100, 285.1) -> (100, 237.6)
  line L1 (100, 237.6) -> (339.6, 237.6)
  line L2 (339.6, 237.6) -> (339.6, 355.6)
  line L3 (339.6, 355.6) -> (-339.6, 355.6)
  line L4 (-339.6, 355.6) -> (-339.6, 237.6)
  line L5 (-339.6, 237.6) -> (-100, 237.6)
  line L6 (-100, 237.6) -> (-100, 285.1)
  arc A0 (-70, 315.1) -> (-100, 285.1) centre (-70, 285.1) ccw
  line L7 (-70, 315.1) -> (70, 315.1)
  arc A1 (100, 285.1) -> (70, 315.1) centre (70, 285.1) ccw
  line L8 (-100, 237.6) -> (-339.6, 237.6)
  line L9 (-339.6, 237.6) -> (-339.6, 257.6)
  line L10 (-339.6, 257.6) -> (-100, 257.6)
  line L11 (-100, 257.6) -> (-100, 237.6)
  line L12 (100, 237.6) -> (339.6, 237.6)
  line L13 (339.6, 237.6) -> (339.6, 257.6)
  line L14 (339.6, 257.6) -> (100, 257.6)
  line L15 (100, 257.6) -> (100, 237.6)
  dimension "d146" = 20
  dimension "d147" = 20
  constraint horizontal L8
  constraint vertical L9
  constraint horizontal L10
  constraint vertical L11
  constraint coincident L4 L9.end
  constraint coincident L5.end L6.start
  constraint horizontal L12
  constraint vertical L13
  constraint horizontal L14
  constraint vertical L15
  constraint coincident L2 L13.end
  constraint coincident L0.end L1.start
  measures "d146" distance of L8 L10
  measures "d147" distance of L12 L14
extrude "Extrude18" add sketch "Sketch16" along normal blind 1 contours L0 L1 L2 L12 L13 L14 L15 | L4 L5 L6 L8 L9 L10 L11 bodies 1
sketch "Sketch17" plane through (-339.6, 0, 0) normal (1, 0, 0) x (0, 1, 0)
  line L0 (583.2, 257.6) -> (584.2, 257.6)
  line L1 (584.2, 257.6) -> (584.2, 355.6)
  line L2 (584.2, 355.6) -> (-584.2, 355.6)
  line L3 (-584.2, 355.6) -> (-584.2, 257.6)
  line L4 (-584.2, 257.6) -> (-583.2, 257.6)
  line L5 (-583.2, 257.6) -> (-583.2, 237.6)
  line L6 (-583.2, 237.6) -> (-5, 237.6)
  line L7 (-5, 237.6) -> (5, 237.6)
  line L8 (5, 237.6) -> (583.2, 237.6)
  line L9 (583.2, 237.6) -> (583.2, 257.6)
  circle A0 centre (217.5, 315.6) radius 8.75
  circle A1 centre (-362.5, 315.6) radius 8.75
  circle A2 centre (-217.5, 315.6) radius 8.75
  circle A3 centre (362.5, 315.6) radius 8.75
  circle A4 centre (72.5, 315.6) radius 8.75
  circle A5 centre (-507.5, 315.6) radius 8.75
  circle A6 centre (-72.5, 315.6) radius 8.75
  circle A7 centre (507.5, 315.6) radius 8.75
  line L10 (-583.2, 257.6) -> (583.2, 257.6)
  line L11 (583.2, 257.6) -> (583.2, 237.6)
  line L12 (583.2, 237.6) -> (-583.2, 237.6)
  line L13 (-583.2, 237.6) -> (-583.2, 257.6)
  constraint horizontal L10
  constraint vertical L11
  constraint horizontal L12
  constraint vertical L13
  constraint coincident L8.end L9.start
  constraint coincident L4.end L5.start
extrude "Extrude19" add sketch "Sketch17" along normal blind 1 contours L5 L6 L7 L8 L9 L10 L11 L12 L13 bodies 1
sketch "Sketch18" plane through (339.6, 0, 0) normal (-1, 0, 0) x (0, -1, 0)
  circle A0 centre (-217.5, 315.6) radius 8.75
  circle A1 centre (362.5, 315.6) radius 8.75
  circle A2 centre (217.5, 315.6) radius 8.75
  circle A3 centre (-362.5, 315.6) radius 8.75
  circle A4 centre (-72.5, 315.6) radius 8.75
  circle A5 centre (507.5, 315.6) radius 8.75
  circle A6 centre (72.5, 315.6) radius 8.75
  circle A7 centre (-507.5, 315.6) radius 8.75
  line L0 (-584.2, 257.6) -> (-583.2, 257.6)
  line L1 (-583.2, 257.6) -> (-583.2, 237.6)
  line L2 (-583.2, 237.6) -> (-5, 237.6)
  line L3 (-5, 237.6) -> (5, 237.6)
  line L4 (5, 237.6) -> (583.2, 237.6)
  line L5 (583.2, 237.6) -> (583.2, 257.6)
  line L6 (583.2, 257.6) -> (584.2, 257.6)
  line L7 (584.2, 257.6) -> (584.2, 355.6)
  line L8 (584.2, 355.6) -> (-584.2, 355.6)
  line L9 (-584.2, 355.6) -> (-584.2, 257.6)
  line L10 (-583.2, 257.6) -> (583.2, 257.6)
  line L11 (583.2, 257.6) -> (583.2, 237.6)
  line L12 (583.2, 237.6) -> (-583.2, 237.6)
  line L13 (-583.2, 237.6) -> (-583.2, 257.6)
  constraint horizontal L10
  constraint vertical L11
  constraint horizontal L12
  constraint vertical L13
  constraint coincident L4.end L5.start
  constraint coincident L0.end L1.start
extrude "Extrude20" add sketch "Sketch18" along normal blind 1 contours L1 L2 L3 L4 L5 L10 L11 L12 L13 bodies 1
sketch "Sketch21" plane through (0, 0, 237.6) normal (0, 0, 1) x (-1, 0, 0)
  line L0 (-338.6, 583.2) -> (-338.6, 5)
  line L1 (-338.6, 5) -> (338.6, 5)
  line L2 (338.6, 5) -> (338.6, 583.2)
  line L3 (338.6, 583.2) -> (90, 583.2)
  line L4 (90, 583.2) -> (90, 673.1)
  line L5 (90, 673.1) -> (-90, 673.1)
  line L6 (-90, 673.1) -> (-90, 583.2)
  line L7 (-90, 583.2) -> (-338.6, 583.2)
  circle A0 centre (0, 0) radius 110
  circle A1 centre (0, 0) radius 100
  dimension "d159" = 220
  dimension "d160" = 200
  constraint coincident A0.centre A1.centre
  constraint concentric A0 A1
  measures "d159" diameter of A0
  measures "d160" diameter of A1
extrude "Extrude22" cut sketch "Sketch21" against normal blind 1 contours L1 A0 A1 | L1 A0 A1 bodies 1
extrude "Extrude23" add 1 faces at (105.9221, -10.2848, 236.6) along direction (0, 0, 1) blind 1 separate body on bodies 1 makes body 2
sketch "Sketch22" plane through (0, 0, 237.6) normal (0, 0, 1) x (-1, 0, 0)
  line L0 (-338.6, -5) -> (-109.8863, -5)
  arc A0 (-109.8863, 5) -> (-109.8863, -5) centre (0, 0) ccw
  circle A1 centre (0, 0) radius 100
  circle A2 centre (0, 0) radius 110
  line L1 (-109.8863, 5) -> (-338.6, 5)
  line L2 (-109.8863, 5) -> (-109.8863, -5)
  line L3 (-109.8863, 5) -> (-338.6, 5)
  line L4 (-338.6, 5) -> (-338.6, -5)
  arc A3 (109.8863, -5) -> (109.8863, 5) centre (0, 0) ccw
  line L5 (109.8863, -5) -> (338.6, -5)
  line L6 (338.6, -5) -> (338.6, 5)
  line L7 (338.6, 5) -> (109.8863, 5)
  line L8 (109.8863, -5) -> (-109.8863, -5)
  line L9 (-109.8863, 5) -> (109.8863, 5)
  dimension "d165" = 200
  dimension "d166" = 220
  constraint concentric A1 A2
  constraint coincident A0.start L1.start
  constraint coincident L1.end L3.end
  constraint coincident L0.end A0.end
  constraint coincident A3.start L5.start
  constraint coincident A3.end L7.end
  measures "d165" diameter of A1
  measures "d166" diameter of A2
extrude "Extrude24" cut sketch "Sketch22" against normal blind 1 contours A1 L8 L9 bodies 1
sketch "Sketch23" plane through (0, 0, 236.6) normal (0, 0, 1) x (-1, 0, 0)
  circle A0 centre (0, 0) radius 100
  line L0 (99.8749, -5) -> (-99.8725, -4.6874)
  line L1 (-99.8723, 4.672) -> (99.8749, 5)
  circle A1 centre (0, 0) radius 110
  arc A2 (99.8749, 5) -> (-99.8749, 5) centre (0, 0) ccw
  line L2 (99.8749, 5) -> (-99.8749, 5)
  line L3 (-99.8749, -5) -> (99.8749, -5)
  arc A3 (-99.8749, -5) -> (99.8749, -5) centre (0, 0) ccw
  dimension "d169" = 200
  constraint concentric A0 A1
  constraint coincident L0.start L3.end
  constraint coincident L1.end A2.start
  measures "d169" diameter of A0
extrude "Extrude25" add sketch "Sketch23" along normal blind 1 separate body contours A0 L2 L3 | A0 A2 L2 | A0 L3 A3 makes body 3
sketch "Sketch24" plane through (0, 0, 237.6) normal (0, 0, 1) x (-1, 0, 0)
  line L0 (338.6, 5) -> (338.6, 583.2)
  line L1 (338.6, 583.2) -> (90, 583.2)
  line L2 (90, 583.2) -> (90, 673.1)
  line L3 (90, 673.1) -> (-90, 673.1)
  line L4 (-90, 673.1) -> (-90, 583.2)
  line L5 (-90, 583.2) -> (-338.6, 583.2)
  line L6 (-338.6, 583.2) -> (-338.6, 5)
  line L7 (130, 458.2) -> (-130, 458.2)
  line L8 (-130, 458.2) -> (-130, 583.2)
  line L9 (-130, 583.2) -> (130, 583.2)
  line L10 (130, 583.2) -> (130, 458.2)
  line L11 (140, 448.2) -> (-140, 448.2)
  line L12 (-140, 448.2) -> (-140, 583.2)
  line L13 (-140, 583.2) -> (140, 583.2)
  line L14 (140, 583.2) -> (140, 448.2)
  line L15 (205, 348.2) -> (-205, 348.2)
  line L16 (-205, 348.2) -> (-205, 583.2)
  line L17 (-205, 583.2) -> (205, 583.2)
  line L18 (205, 583.2) -> (205, 348.2)
  line L19 (215, 338.2) -> (-215, 338.2)
  line L20 (-215, 338.2) -> (-215, 583.2)
  line L21 (-215, 583.2) -> (215, 583.2)
  line L22 (215, 583.2) -> (215, 338.2)
  circle A0 centre (0, 203.2) radius 10
  circle A1 centre (0, -203.2) radius 10
  line L23 (130, -583.2) -> (-130, -583.2)
  line L24 (-130, -583.2) -> (-130, -458.2)
  line L25 (-130, -458.2) -> (130, -458.2)
  line L26 (130, -458.2) -> (130, -583.2)
  line L27 (140, -583.2) -> (-140, -583.2)
  line L28 (-140, -583.2) -> (-140, -448.2)
  line L29 (-140, -448.2) -> (140, -448.2)
  line L30 (140, -448.2) -> (140, -583.2)
  line L31 (205, -583.2) -> (-205, -583.2)
  line L32 (-205, -583.2) -> (-205, -348.2)
  line L33 (-205, -348.2) -> (205, -348.2)
  line L34 (205, -348.2) -> (205, -583.2)
  line L35 (215, -583.2) -> (-215, -583.2)
  line L36 (-215, -583.2) -> (-215, -338.2)
  line L37 (-215, -338.2) -> (215, -338.2)
  line L38 (215, -338.2) -> (215, -583.2)
  arc A2 (109.8863, 5) -> (-109.8863, 5) centre (0, 0) ccw
  line L39 (109.8863, 5) -> (338.6, 5)
  line L40 (-338.6, 5) -> (-109.8863, 5)
  circle A3 centre (0, 378.2) radius 67.5
  circle A4 centre (0, 378.2) radius 77.5
  circle A5 centre (0, -378.2) radius 67.5
  circle A6 centre (0, -378.2) radius 77.5
  point P0 (90, -583.2)
  dimension "d174" = 10
  dimension "d175" = 10
  dimension "d176" = 10
  dimension "d177" = 125
  dimension "d178" = 100
  dimension "d179" = 65
  dimension "d180" = 65
  dimension "d181" = 10
  dimension "d182" = 10
  dimension "d183" = 10
  dimension "d187" = 20
  dimension "d189" = 20
  dimension "d191" = 10
  dimension "d192" = 10
  dimension "d193" = 100
  dimension "d194" = 125
  dimension "d208" = 260
  dimension "d209" = 130
  dimension "d211" = 135
  dimension "d215" = 135
  dimension "d216" = 155
  dimension "d217" = 135
  dimension "d218" = 135
  dimension "d219" = 155
  dimension "d220" = 175
  dimension "d221" = 175
  constraint horizontal L7
  constraint vertical L8
  constraint horizontal L9
  constraint vertical L10
  constraint coincident L5 L8.end
  constraint horizontal L11
  constraint vertical L12
  constraint horizontal L13
  constraint vertical L14
  constraint coincident L5 L12.end
  constraint horizontal L15
  constraint vertical L16
  constraint horizontal L17
  constraint vertical L18
  constraint coincident L5 L16.end
  constraint horizontal L19
  constraint vertical L20
  constraint horizontal L21
  constraint vertical L22
  constraint coincident L5 L20.end
  constraint vertical A2.centre A0.centre
  constraint vertical A2.centre A1.centre
  constraint horizontal L23
  constraint vertical L24
  constraint horizontal L25
  constraint vertical L26
  constraint horizontal L23.start P0
  constraint horizontal L27
  constraint vertical L28
  constraint horizontal L29
  constraint vertical L30
  constraint horizontal P0 L27.start
  constraint horizontal L31
  constraint vertical L32
  constraint horizontal L33
  constraint vertical L34
  constraint horizontal L35
  constraint vertical L36
  constraint horizontal L37
  constraint vertical L38
  constraint horizontal P0 L35.start
  constraint horizontal P0 L31.start
  constraint vertical L7.start L25.end
  constraint vertical L11.start L29.end
  constraint vertical L7.end L24.end
  constraint vertical L11.end L28.end
  constraint vertical L15.start L33.end
  constraint vertical L19.start L37.end
  constraint vertical L15.end L32.end
  constraint vertical L19.end L36.end
  constraint concentric A3 A4
  constraint vertical A2.centre A3.centre
  constraint concentric A5 A6
  constraint vertical A2.centre A5.centre
  measures "d174" distance of L10 L14
  measures "d175" distance of L8 L12
  measures "d176" distance of L7 L11
  measures "d177" distance of L7 L9
  measures "d178" distance of L11 L15
  measures "d179" distance of L14 L18
  measures "d180" distance of L12 L16
  measures "d181" distance of L15 L19
  measures "d182" distance of L16 L20
  measures "d183" distance of L18 L22
  measures "d187" diameter of A0
  measures "d189" diameter of A1
  measures "d191" distance of L25 L29
  measures "d192" distance of L33 L37
  measures "d193" distance of L29 L33
  measures "d194" distance of L23 L25
  measures "d208" distance of L8 L10
  measures "d209" distance of A2.centre L8
  measures "d211" distance of L19 A0.centre
  measures "d215" diameter of A3
  measures "d216" diameter of A4
  measures "d217" distance of A1.centre L37
  measures "d218" diameter of A5
  measures "d219" diameter of A6
  measures "d220" distance of A1.centre A5.centre
  measures "d221" distance of A0.centre A3.centre
extrude "Extrude29" cut sketch "Sketch24" against normal blind 1 contours L1 L15 L18 L19 L21 L22 A4 | L1 L5 L7 L8 L10 L11 L12 L13 L14 L17 L21 A4 | L19 A3 A4 | L15 L19 A3 A4 | L15 L19 A3 | L15 L19 A3 A4 | L5 L15 L16 L19 L20 L21 A4 | L11 A4 | A0 | A1 | L24 L25 L26 L27 L28 L29 L30 L31 L35 A6 | L33 L34 L35 L37 L38 A6 | L32 L33 L35 L36 L37 A6 | L29 A6 | L33 L37 A5 A6 | L33 L37 A5 A6 | L33 L37 A5 | L37 A5 A6 bodies 1
extrude "Extrude30" add 6 faces at (43.3333, 451.5333, 236.6) (-22.1265, 344.8667, 236.6) (-3.0405, 205.1431, 236.6) (22.1265, -344.8667, 236.6) (-43.3333, -451.5333, 236.6) (-3.0405, -201.2569, 236.6) along direction (0, 0, 1) blind 1 separate body on bodies 1 makes body 4 at (-43.3333, -451.5333, 236.6) makes body 5 at (-3.0405, 205.1431, 236.6) makes body 6 at (43.3333, 451.5333, 236.6) makes body 7 at (-22.1265, 344.8667, 236.6) makes body 8 at (22.1265, -344.8667, 236.6) makes body 9 at (-3.0405, -201.2569, 236.6)
sketch "Sketch26" plane through (0, 0, 237.6) normal (0, 0, 1) x (-1, 0, 0)
  circle A0 centre (0, 203.2) radius 10
  line L0 (215, 583.2) -> (215, 338.2)
  line L1 (215, 338.2) -> (66.3796, 338.2)
  arc A1 (-66.3796, 338.2) -> (66.3796, 338.2) centre (0, 378.2) ccw
  line L2 (-66.3796, 338.2) -> (-215, 338.2)
  line L3 (-215, 338.2) -> (-215, 583.2)
  line L4 (-215, 583.2) -> (-338.6, 583.2)
  line L5 (-338.6, 583.2) -> (-338.6, 5)
  line L6 (-338.6, 5) -> (-109.8863, 5)
  arc A2 (109.8863, 5) -> (-109.8863, 5) centre (0, 0) ccw
  line L7 (109.8863, 5) -> (338.6, 5)
  line L8 (338.6, 5) -> (338.6, 583.2)
  line L9 (338.6, 583.2) -> (215, 583.2)
  line L10 (105, 583.2) -> (338.6, 348.2)
  line L11 (338.6, 583.2) -> (105, 583.2)
  line L12 (-338.6, 583.2) -> (-338.6, 348.2)
  line L13 (-105, 583.2) -> (-338.6, 583.2)
  line L14 (-105, 583.2) -> (-338.6, 348.2)
  line L15 (338.6, -583.2) -> (338.6, -348.2)
  line L16 (338.6, -348.2) -> (338.6, -572.8458)
  line L17 (338.6, -572.8458) -> (338.6, -583.2)
  line L18 (338.6, -348.2) -> (105, -583.2)
  line L19 (338.6, -583.2) -> (105, -583.2)
  line L20 (-105, -583.2) -> (-338.6, -583.2)
  line L21 (-338.6, -583.2) -> (-338.6, -348.2)
  line L22 (-338.6, -348.2) -> (-105, -583.2)
  point P0 (100, 583.2)
  point P1 (205, 348.2)
  point P2 (-205, 348.2)
  point P3 (-100, 583.2)
  point P4 (338.6, -583.2)
  point P5 (90, -583.2)
  point P6 (100, -583.2)
  point P7 (205, -348.2)
  point P8 (-100, -583.2)
  point P9 (-205, -348.2)
  dimension "d226" = 5
  dimension "d227" = 5
  dimension "d228" = 5
  dimension "d229" = 5
  constraint coincident L8 L10.end
  constraint coincident L8.end L9.start
  constraint perpendicular L8 L11
  constraint horizontal L10.end P1
  constraint coincident L4.end L5.start
  constraint coincident L5 L12.end
  constraint perpendicular L5 L13
  constraint horizontal L12.end P2
  constraint vertical L15
  constraint vertical L8.end P4
  constraint vertical L16
  constraint coincident P4 L15.start
  constraint horizontal L18.end P5
  constraint horizontal L15.end P7
  constraint horizontal L20
  constraint vertical L12.end L21.end
  constraint vertical L4.end L20.end
  constraint horizontal P4 L20.end
  constraint horizontal L21.end P9
  measures "d226" distance of L10.start P0
  measures "d227" distance of L13.start P3
  measures "d228" distance of L18.end P6
  measures "d229" distance of L20.start P8